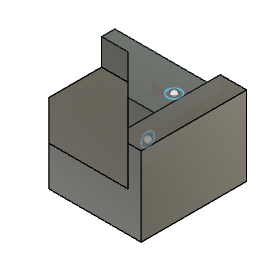
Shape 1_ (Autodesk Fusion 360 design; units mm, degrees)
Autodesk Fusion 360 part; units mm, degrees
sketch "Sketch1" plane through (0, 0, 0) normal (0, 0, 1) x (1, 0, 0)
  line L0 (0, 0) -> (-140, 0)
  line L1 (-140, 0) -> (-140, -160)
  line L2 (-140, -160) -> (0, -160)
  line L3 (0, -160) -> (0, 0)
  dimension "d1" = 140
  dimension "d2" = 160
  constraint horizontal L0
  constraint vertical L1
  constraint horizontal L2
  constraint vertical L3
  constraint coincident L0.start L3.end
  measures "d1" distance of L0.start L0.end
  measures "d2" distance of L0.start L2.end
extrude "Extrude1" add sketch "Sketch1" along normal blind 60
sketch "Sketch2" plane through (0, 0, 0) normal (0, 0, 1) x (1, 0, 0)
  line L0 (-140, 0) -> (-200, 0)
  line L1 (-200, 0) -> (-200, -100)
  line L2 (-200, -100) -> (-140, -100)
  line L3 (-140, -100) -> (-140, 0)
  dimension "d5" = 60
  dimension "d6" = 100
  constraint horizontal L0
  constraint vertical L1
  constraint horizontal L2
  constraint vertical L3
  measures "d5" distance of L0.start L0.end
  measures "d6" distance of L0.start L2.end
extrude "Extrude2" add sketch "Sketch2" along normal blind 60
sketch "Sketch3" plane through (0, 0, 0) normal (0, 0, 1) x (1, 0, 0)
sketch "Sketch4" plane through (0, 0, 0) normal (0, 0, 1) x (1, 0, 0)
  line L0 (-140, -160) -> (-200, -100)
  line L1 (-200, -100) -> (-140, -100)
  line L2 (-140, -100) -> (-140, -160)
  constraint horizontal L1
  constraint perpendicular L1 L2
extrude "Extrude3" add sketch "Sketch4" along normal blind 60
sketch "Sketch5" plane through (0, 0, 60) normal (0, 0, 1) x (-1, 0, 0)
  line L0 (0, 160) -> (0, 0)
  line L1 (0, 0) -> (200, 0)
  line L2 (200, 0) -> (200, 100)
  line L3 (200, 100) -> (140, 160)
  line L4 (140, 160) -> (0, 160)
  line L5 (0, 0) -> (20, 0)
  line L6 (20, 0) -> (20, 160)
  line L7 (20, 160) -> (0, 160)
  line L8 (0, 160) -> (0, 0)
  dimension "d11" = 20
  constraint horizontal L5
  constraint vertical L6
  constraint horizontal L7
  constraint vertical L8
  constraint coincident L0.end L1.start
  measures "d11" distance of L0.end L5.end
extrude "Extrude4" add sketch "Sketch5" along normal blind 60 contours L0 L1 L4 L5 L6 L7 L8
sketch "Sketch6" plane through (0, 0, 60) normal (0, 0, 1) x (-1, 0, 0)
  line L0 (20, 160) -> (20, 0)
  line L1 (20, 0) -> (200, 0)
  line L2 (200, 0) -> (200, 100)
  line L3 (200, 100) -> (140, 160)
  line L4 (140, 160) -> (20, 160)
  line L5 (20, 0) -> (40, 0)
  line L6 (40, 0) -> (40, 140)
  line L7 (40, 140) -> (20, 140)
  line L8 (20, 140) -> (20, 0)
  dimension "d14" = 20
  dimension "d15" = 140
  constraint horizontal L5
  constraint vertical L6
  constraint horizontal L7
  constraint vertical L8
  constraint coincident L0.end L1.start
  measures "d14" distance of L0.end L5.end
  measures "d15" distance of L0.end L7.end
extrude "Extrude5" add sketch "Sketch6" along normal blind 60 contours L0 L1 L5 L6 L7 L8
sketch "Sketch7" plane through (0, 0, 60) normal (0, 0, 1) x (-1, 0, 0)
  line L0 (20, 140) -> (40, 140)
  line L1 (40, 140) -> (40, 0)
  line L2 (40, 0) -> (200, 0)
  line L3 (200, 0) -> (200, 100)
  line L4 (200, 100) -> (140, 160)
  line L5 (140, 160) -> (20, 160)
  line L6 (20, 160) -> (20, 140)
  line L7 (40, 140) -> (20, 160)
  line L8 (20, 140) -> (40, 140)
  constraint coincident L0.end L1.start
  constraint coincident L5.end L6.start
  constraint coincident L0.start L6.end
extrude "Extrude6" add sketch "Sketch7" along normal blind 60 contours L0 L6 L7 L8
sketch "Sketch8" plane through (0, 0, 60) normal (0, 0, 1) x (-1, 0, 0)
  line L0 (20, 160) -> (40, 140)
  line L1 (40, 140) -> (40, 0)
  line L2 (40, 0) -> (200, 0)
  line L3 (200, 0) -> (200, 100)
  line L4 (200, 100) -> (140, 160)
  line L5 (140, 160) -> (20, 160)
  line L6 (40, 0) -> (100, 0)
  line L7 (100, 0) -> (100, 80)
  line L8 (100, 80) -> (40, 80)
  line L9 (40, 80) -> (40, 0)
  dimension "d20" = 60
  dimension "d21" = 80
  constraint horizontal L6
  constraint vertical L7
  constraint horizontal L8
  constraint vertical L9
  constraint coincident L1.end L2.start
  measures "d20" distance of L1.end L6.end
  measures "d21" distance of L1.end L8.end
extrude "Extrude7" add sketch "Sketch8" along normal blind 40 contours L1 L2 L6 L7 L8 L9
sketch "Sketch9" plane through (0, 0, 60) normal (0, 0, 1) x (-1, 0, 0)
  line L0 (100, 80) -> (100, 0)
  line L1 (100, 0) -> (200, 0)
  line L2 (200, 0) -> (200, 100)
  line L3 (200, 100) -> (140, 160)
  line L4 (140, 160) -> (20, 160)
  line L5 (20, 160) -> (40, 140)
  line L6 (40, 140) -> (40, 80)
  line L7 (40, 80) -> (100, 80)
  line L8 (200, 0) -> (160, 0)
  line L9 (160, 0) -> (160, 20)
  line L10 (160, 20) -> (200, 20)
  line L11 (200, 20) -> (200, 0)
  dimension "d24" = 40
  dimension "d25" = 20
  constraint horizontal L8
  constraint vertical L9
  constraint horizontal L10
  constraint vertical L11
  constraint coincident L1.end L2.start
  measures "d24" distance of L1.end L8.end
  measures "d25" distance of L1.end L10.end
extrude "Extrude8" add sketch "Sketch9" along normal blind 40 contours L1 L2 L8 L9 L10 L11
sketch "Sketch10" plane through (0, 0, 60) normal (0, 0, 1) x (-1, 0, 0)
  line L0 (160, 0) -> (160, 20)
  line L1 (160, 20) -> (200, 20)
  line L2 (200, 20) -> (200, 100)
  line L3 (200, 100) -> (140, 160)
  line L4 (140, 160) -> (20, 160)
  line L5 (20, 160) -> (40, 140)
  line L6 (40, 140) -> (40, 80)
  line L7 (40, 80) -> (100, 80)
  line L8 (100, 80) -> (100, 0)
  line L9 (100, 0) -> (160, 0)
  line L10 (160, 20) -> (160, 0)
  line L11 (100, 0) -> (100, 80)
  line L12 (160, 20) -> (100, 80)
  constraint coincident L0.end L1.start
  constraint coincident L0.start L9.end
  constraint coincident L8.end L9.start
  constraint coincident L7.end L8.start
extrude "Extrude9" add sketch "Sketch10" along normal blind 40 contours L0 L8 L9 L10 L11 L12
sketch "Sketch11" plane through (-40, 0, 0) normal (-1, 0, 0) x (0, -1, 0)
  line L0 (0, 100) -> (80, 100)
  line L1 (80, 100) -> (80, 60)
  line L2 (80, 60) -> (140, 60)
  line L3 (140, 60) -> (140, 120)
  line L4 (140, 120) -> (0, 120)
  line L5 (0, 120) -> (0, 100)
sketch "Sketch12" plane through (-40, -70, 90) normal (-1, 0, 0) x (0, -1, 0)
  circle A0 centre (40, 0) radius 10
  dimension "d31" = 20
  measures "d31" diameter of A0
sketch "Sketch13" plane through (0, 0, 100) normal (0, 0, 1) x (-1, 0, 0)
  line L0 (40, 80) -> (40, 0)
  line L1 (40, 0) -> (200, 0)
  line L2 (200, 0) -> (200, 20)
  line L3 (200, 20) -> (160, 20)
  line L4 (160, 20) -> (100, 80)
  line L5 (100, 80) -> (40, 80)
  circle A0 centre (70, 40) radius 10
  dimension "d34" = 20
  measures "d34" diameter of A0
